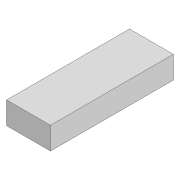
# Autodesk Inventor part: 3s lipo battery
Saved by Autodesk Inventor 2022 (Build 260153000, 153)
## iProperties
Created: 2024-06-11
Part Number: 3s lipo battery
Material: Generic
Document SubType Name: Modeling
Designer: david
Density: 1 g/cm^3
Appearance: Default
Author: david
Autodesk Inventor part; units mm, degrees
ref_plane "YZ Plane" through (0, 0, 0) normal (1, 0, 0) x (0, 1, 0)
ref_plane "XZ Plane" through (0, 0, 0) normal (0, 1, 0) x (-1, 0, 0)
ref_plane "XY Plane" through (0, 0, 0) normal (0, 0, 1) x (1, 0, 0)
sketch "Sketch1" plane through (0, 0, 0) normal (0, 0, 1) x (1, 0, 0)
  line L0 (-25.5, -13) -> (25.5, -13)
  line L1 (25.5, -13) -> (25.5, 13)
  line L2 (25.5, 13) -> (-25.5, 13)
  line L3 (-25.5, 13) -> (-25.5, -13)
  line L4 (-25.5, -13) -> (25.5, 13) construction
  line L5 (25.5, -13) -> (-25.5, 13) construction
  point P0 (0, 0)
  dimension "d0" = 51
  dimension "d1" = 26
  constraints: 12 end point, 2 midpoint, 2 parallel, 1 horizontal, 1 perpendicular
  measures "d0" distance of L1.end L2.end
  measures "d1" distance of L0.end L1.end
extrude "Lipo Body" add sketch "Sketch1" against normal blind 143
body "Solid1"
